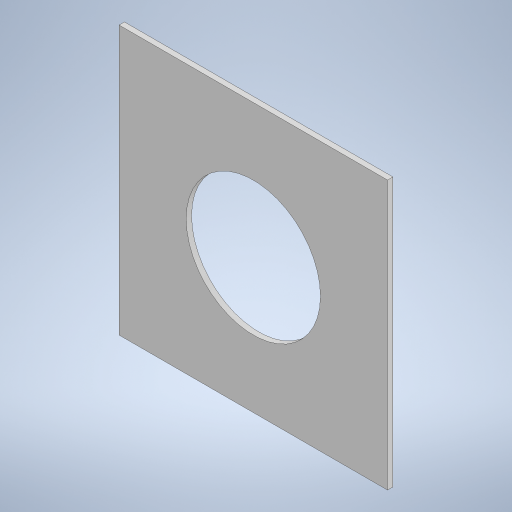
# Autodesk Inventor part: Part5
Saved by Autodesk Inventor 2024 (Build 280153000, 153)
## iProperties
Created: 2023-10-19
Part Number: Part5
Material: Generic
Document SubType Name: Modeling
Designer: liuyu
Density: 1 g/cm^3
Appearance: Default
Author: liuyu
Autodesk Inventor part; units mm, degrees
ref_plane "YZ Plane" through (0, 0, 0) normal (1, 0, 0) x (0, 1, 0)
ref_plane "XZ Plane" through (0, 0, 0) normal (0, 1, 0) x (-1, 0, 0)
ref_plane "XY Plane" through (0, 0, 0) normal (0, 0, 1) x (1, 0, 0)
sketch "Sketch1" plane through (0, 0, 0) normal (0, 0, 1) x (1, 0, 0)
  line L0 (-12.331, 15.8004) -> (-262.331, 15.8004)
  line L1 (-262.331, 15.8004) -> (-262.331, -234.1996)
  line L2 (-262.331, -234.1996) -> (-12.331, -234.1996)
  line L3 (-12.331, -234.1996) -> (-12.331, 15.8004)
  circle A0 centre (-137.331, -109.1996) radius 62.5
  point P0 (0, 0)
  dimension "d0" = 250
  dimension "d1" = 250
  dimension "d2" = 125
  constraints: 8 end point, 2 parallel, 1 centre point, 1 horizontal, 1 perpendicular
  measures "d0" distance of L2.end L1.end
  measures "d1" distance of L1.end L0.end
  measures "d2" diameter of A0
extrude "Extrusion1" add sketch "Sketch1" along normal blind 5
body "Solid1"
